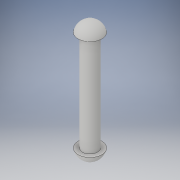
# Autodesk Inventor part: rebite garra
Saved by Autodesk Inventor 2017 (Build 210142000, 142)
## iProperties
Part Number: rebite garra
Material: Genérico
Document SubType Name: Modeling
Designer: jorda
Density: 1 g/cm^3
Appearance: Padrão
Author: jorda
Autodesk Inventor part; units mm, degrees
ref_plane "YZ Plane" through (0, 0, 0) normal (1, 0, 0) x (0, 1, 0)
ref_plane "XZ Plane" through (0, 0, 0) normal (0, 1, 0) x (-1, 0, 0)
ref_plane "XY Plane" through (0, 0, 0) normal (0, 0, 1) x (1, 0, 0)
sketch "Esboço1" plane through (0, 0, 0) normal (1, 0, 0) x (0, 1, 0)
  arc A0 (4.7149, 0.9) -> (0, 4.8) centre (0, 0) ccw
  line L0 (0, 0.9) -> (4.7149, 0.9)
  line L1 (0, 0.9) -> (0, 4.8)
  constraints: 4 end point, 2 point on circle, 1 centre point, 1 horizontal
revolve "Revolução1" add sketch "Esboço1" angle 360 about axis through (0, 0, 0.9) along (0, 0, 1)
sketch "Esboço2" plane through (0, 0, 0.9) normal (0, 0, -1) x (-1, 0, 0)
  circle A0 centre (0, 0) radius 3
  dimension "d4" = 6
  constraints: 1 centre point, 1 coincident
  measures "d4" diameter of A0
extrude "Extrusão1" add sketch "Esboço2" along normal blind 40
ref_plane "Work Plane1" through (0, 0, -19.1) normal (0, 0, -1) x (-1, 0, 0)
mirror "Mirror1" about plane through (0, 0, -19.1) normal (0, 0, -1) of "Revolução1"
